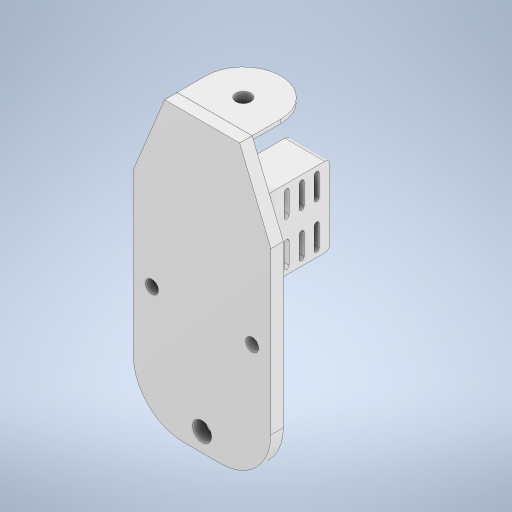
# Autodesk Inventor part: Electromagnet Gantry Plate
Saved by Autodesk Inventor 2023.2 (Build 272271030, 271C)
## iProperties
Created: 2023-04-10
Part Number: Electromagnet Gantry Plate
Material: PC/ABS Plastic
Document SubType Name: Modeling
Designer: ethan
Density: 0.357273 g/cm^3
Appearance: Smooth - White
Author: ethan
Autodesk Inventor part; units mm, degrees
ref_plane "YZ Plane" through (0, 0, 0) normal (1, 0, 0) x (0, 1, 0)
ref_plane "XZ Plane" through (0, 0, 0) normal (0, 1, 0) x (-1, 0, 0)
ref_plane "XY Plane" through (0, 0, 0) normal (0, 0, 1) x (1, 0, 0)
sketch "Sketch1" plane through (0, 0, 0) normal (0, 1, 0) x (-1, 0, 0)
  line L0 (0, 0) -> (55, 0)
  line L1 (55, 0) -> (55, -55)
  line L2 (55, -55) -> (0, -55)
  line L3 (0, -55) -> (0, 0)
  line L4 (47.55, -7.45) -> (7.45, -7.45) construction
  line L5 (7.45, -7.45) -> (7.45, -47.55) construction
  line L6 (7.45, -47.55) -> (47.55, -47.55) construction
  line L7 (47.55, -47.55) -> (47.55, -7.45) construction
  circle A0 centre (47.55, -7.45) radius 2.6
  circle A1 centre (47.55, -47.55) radius 2.6
  circle A2 centre (7.45, -47.55) radius 2.6
  circle A3 centre (7.45, -7.45) radius 2.6
  circle A4 centre (47.55, -7.45) radius 12.5 construction
  circle A5 centre (27.5, -7.45) radius 3.8
  line L8 (55, -55) -> (0, -55)
  line L9 (0, -55) -> (0, -139.9)
  line L10 (0, -139.9) -> (55, -139.9)
  line L11 (55, -139.9) -> (55, -55)
  point P0 (3.72, -55)
  dimension "d0" = 55
  dimension "d1" = 55
  dimension "d2" = 40.1
  dimension "d3" = 40.1
  dimension "d4" = 5.2
  dimension "d5" = 5.2
  dimension "d6" = 5.2
  dimension "d7" = 5.2
  dimension "d8" = 7.45
  dimension "d9" = 7.45
  dimension "d13" = 25
  dimension "d78" = 7.6
  dimension "d160" = 84.9
  constraints: 24 end point, 6 centre point, 6 parallel, 5 coincident, 3 horizontal, 3 perpendicular, 1 midpoint
  measures "d0" distance of L1.end L2.end
  measures "d1" distance of L0.end L1.end
  measures "d2" distance of L6.end L5.end
  measures "d3" distance of L5.end L4.end
  measures "d4" diameter of A0
  measures "d5" diameter of A3
  measures "d6" diameter of A1
  measures "d7" diameter of A2
  measures "d8" distance between parallel lines of L1 L7
  measures "d9" distance from line of L2 L5.end
  measures "d13" diameter of A4
  measures "d78" diameter of A5
  measures "d160" distance of L2.end L9.end
extrude "Extrusion1" add sketch "Sketch1" along normal blind 5 contours L0 L1 L2 L3 | L2 L11 L10 L9 | A0 | A3
fillet "Fillet1" radius 20 2 edges at (-55, 2.5, 0) (0, 2.5, 0)
ref_plane "Work Plane14" through (0, 0, 0) normal (0, 1, 0) x (1, 0, 0)
sketch "Sketch7" plane through (0, 0, 0) normal (0, 1, 0) x (1, 0, 0)
  line L0 (-19.45, 63) -> (-19.45, 55)
  line L1 (-35.55, 19.45) -> (-35.55, 63) projected
  line L2 (-19.45, 55) -> (-35.55, 55)
  line L3 (-35.55, 55) -> (-35.55, 63)
  line L4 (-35.55, 63) -> (-19.45, 63)
  line L5 (-19.45, 63) -> (-19.45, 55)
  circle A0 centre (-47.55, 47.55) radius 2.6 projected
  circle A1 centre (-47.55, 47.55) radius 12
  circle A2 centre (-7.45, 47.55) radius 2.6 projected
  circle A3 centre (-7.45, 47.55) radius 12
  point P0 (0, 0)
  point P1 (-53, 55)
  dimension "d67" = 24
  dimension "d68" = 24
  constraints: 10 end point, 2 centre point, 2 coincident, 2 parallel, 1 horizontal, 1 perpendicular
  measures "d67" diameter of A1
  measures "d68" diameter of A3
extrude "Extrusion9" add sketch "Sketch7" along normal blind 25 contours L0 L2 L1 L4
ref_plane "Work Plane2" through (-19.45, -5, -63) normal (0, 0, -1) x (-1, 0, 0)
sketch "Sketch9" plane through (-19.45, -5, -63) normal (0, 0, -1) x (-1, 0, 0)
  line L0 (0, 0) -> (0, 8) projected
  line L1 (16.1, 8) -> (16.1, 5) projected
  line L2 (0, 8) -> (16.1, 8)
  line L3 (4.55, 8) -> (11.55, 8) projected
  line L4 (8.05, 8) -> (8.05, 21.475)
  circle A0 centre (8.05, 21.475) radius 3
  point P0 (-19.45, 5)
  dimension "d54" = 13.475
  dimension "d55" = 6
  constraints: 4 end point, 1 centre point, 1 coincident, 1 midpoint, 1 perpendicular, 1 vertical
  measures "d54" distance of L4.start L4.end
  measures "d55" diameter of A0
extrude "Extrusion11" cut sketch "Sketch9" against normal through all
ref_plane "Work Plane12" through (-19.45, 0, -63) normal (0, 0, -1) x (-1, 0, 0)
sketch "Sketch10" plane through (-19.45, 0, -63) normal (0, 0, -1) x (-1, 0, 0)
  circle A0 centre (8.05, 16.475) radius 3 projected
  arc A1 (23.05, 16.475) -> (-6.95, 16.475) centre (8.05, 16.475) ccw
  line L0 (-6.95, 16.475) -> (-6.95, 0)
  line L1 (23.05, 16.475) -> (23.05, 0)
  line L2 (-6.95, 0) -> (23.05, 0)
  line L3 (33.55, 0) -> (-17.45, 0) projected
  point P0 (-19.45, 0)
  dimension "d60" = 30
  constraints: 6 end point, 2 point on circle, 2 tangent, 2 vertical, 1 centre point, 1 coincident, 1 collinear
  measures "d60" diameter of A1
extrude "Extrusion12" add sketch "Sketch10" against normal up to surface (8 mm away)
sketch "Sketch18" plane through (0, 5, 0) normal (0, 1, 0) x (1, 0, 0)
  circle A0 centre (-47.55, 47.55) radius 2.6 projected
  circle A1 centre (-47.55, 47.55) radius 12 construction
  line L0 (-47.55, 37.5) -> (0, 37.5)
  line L1 (0, 20) -> (0, 139.9) projected
  line L2 (-47.55, 54.5) -> (0, 54.5)
  line L3 (-47.55, 63) -> (0, 63)
  line L4 (-47.55, 72) -> (0, 72)
  line L5 (-47.55, 80.5) -> (0, 80.5)
  line L6 (-47.55, 139.9) -> (0, 139.9)
  point P0 (0, 0)
  point P1 (0, 63)
  point P2 (0, 83)
  dimension "d106" = 24
  dimension "d107" = 10.05
  dimension "d108" = 17
  dimension "d109" = 8.5
  dimension "d110" = 34.5
  dimension "d111" = 8.5
  dimension "d206" = 102.4
  constraints: 12 end point, 5 parallel, 1 centre point, 1 coincident, 1 horizontal, 1 point on line
  measures "d106" diameter of A1
  measures "d107" distance of A0.centre L0.start
  measures "d108" distance between parallel lines of L0 L2
  measures "d109" distance between parallel lines of L2 L3
  measures "d110" distance between parallel lines of L0 L4
  measures "d111" distance between parallel lines of L4 L5
  measures "d206" distance between parallel lines of L0 L6
ref_plane "Work Plane10" through (-27.5, 0, -20) normal (-1, 0, 0) x (0, 0, 1)
chamfer "Chamfer5" distance 6.5 angle 45 3 edges at (-27.5, 31.475, -55) (-42.5, 10.7375, -55) (-12.5, 10.7375, -55)
chamfer "Chamfer6" distance 6 angle 45 1 edges at (-27.5, 5, -55)
ref_plane "Work Plane16" through (0, 0, -114.9) normal (0, 0, -1) x (-1, 0, 0)
move faces "Move1" translate (0, 0, -51.9) faces at (-27.6205, 7.8323, -63) (-12.6942, 18.8812, -62.5) (-42.5, 8.825, -62.5) (-40.3333, 10.825, -59.3333) (-39.1188, 18.2262, -58.25) (-14.6667, 10.825, -59.3333) (-12.5, 8.825, -62) (-27.6205, 11.8323, -55) (-26.6667, 9, -53) (-30.4903, 16.2336, -57.6667)
sketch "Sketch29" plane through (0, 5, 0) normal (0, 1, 0) x (1, 0, 0)
  line L0 (0, 139.9) -> (-55, 139.9) projected
  line L1 (0, 20) -> (0, 139.9) projected
  line L2 (-55, 139.9) -> (0, 139.9)
  line L3 (0, 139.9) -> (0, 114.877)
  line L4 (0, 114.877) -> (-55, 114.877)
  line L5 (-55, 114.877) -> (-55, 139.9)
  line L6 (-42.5, 114.9) -> (-42.5, 113.4) projected
  line L7 (-50, 84.5) -> (-55, 84.5) projected
  line L8 (-42.5, 114.9) -> (-55, 84.5)
  line L9 (-55, 84.5) -> (-55, 114.877)
  line L10 (-12.5, 114.9) -> (-12.5, 113.4) projected
  line L11 (-12.5, 114.9) -> (0, 84.5)
  line L12 (0, 84.5) -> (0, 114.877)
  line L13 (0, 20) -> (0, 139.9) projected
  point P0 (0, 0)
  point P1 (-42.5, 114.877)
  point P2 (-12.5, 114.877)
  constraints: 16 end point, 2 parallel, 2 perpendicular, 1 collinear, 1 horizontal, 1 point on line
extrude "Extrusion31" cut sketch "Sketch29" against normal through all contours L1 L4 L11 L10 L6 L8 L5 L0 | L1 L11 L4 | L4 L8 L9
sketch "Sketch31" plane through (0, 5, 0) normal (0, 1, 0) x (1, 0, 0)
  circle A0 centre (-47.55, 47.55) radius 2.6 projected
  circle A1 centre (-7.45, 47.55) radius 2.6 projected
  line L0 (-47.55, 47.55) -> (-7.45, 47.55)
  line L1 (-27.5, 47.55) -> (-27.5, 80.5)
  line L2 (-33.5, 47.55) -> (-33.5, 80.5)
  line L3 (-21.5, 47.55) -> (-21.5, 80.5)
  line L4 (-33.5, 80.5) -> (-21.5, 80.5)
  line L5 (-33.5, 47.55) -> (-21.5, 47.55)
  line L6 (-19.5, 84.5) -> (-19.5, 44.7007)
  line L7 (-19.5, 44.7007) -> (-35.5, 44.7007)
  line L8 (-35.5, 44.7007) -> (-35.5, 84.5)
  line L9 (-35.5, 84.5) -> (-19.5, 84.5)
  point P0 (0, 0)
  point P1 (-19.5, 82.5)
  point P2 (-35.5, 81.6507)
  dimension "d216" = 32.95
  dimension "d217" = 6
  dimension "d218" = 6
  dimension "d225" = 2
  dimension "d231" = 4
  constraints: 20 end point, 3 horizontal, 2 parallel, 2 point on line, 1 collinear, 1 midpoint, 1 vertical
  measures "d216" distance of L1.start L1.end
  measures "d217" distance between parallel lines of L1 L2
  measures "d218" distance between parallel lines of L1 L3
  measures "d225" distance between parallel lines of L3 L6
  measures "d231" distance between parallel lines of L4 L9
extrude "Extrusion32" add sketch "Sketch31" along normal blind 38.1 contours L2 L4 L1 L0 | L0 L6 L7 L8 | L0 L8 L9 L6 L3 L4 L2 | L1 L4 L3 L0
sketch "Sketch34" plane through (-35.5, 5, -84.5) normal (-1, 0, 0) x (0, 0, 1)
  line L0 (0, 38.1) -> (39.7993, 38.1) projected
  line L1 (39.7993, 0) -> (39.7993, 38.1) projected
  line L2 (39.7993, 38.1) -> (39.7993, 0)
  line L3 (35.7993, 0) -> (35.7993, 38.1)
  line L4 (28.8493, 0) -> (28.8493, 38.1)
  line L5 (20.3493, 0) -> (20.3493, 38.1)
  line L6 (11.3493, 0) -> (11.3493, 38.1)
  line L7 (2.8493, 0) -> (2.8493, 38.1)
  line L8 (2.8493, 32.8026) -> (11.3493, 32.8026) construction
  line L9 (2.8493, 31.8026) -> (11.3493, 31.8026)
  line L10 (11.3493, 33.8026) -> (2.8493, 33.8026)
  arc A0 (2.8493, 33.8026) -> (2.8493, 31.8026) centre (2.8493, 32.8026) ccw
  arc A1 (11.3493, 31.8026) -> (11.3493, 33.8026) centre (11.3493, 32.8026) ccw
  line L11 (20.3493, 32.8026) -> (28.8493, 32.8026) construction
  line L12 (20.3493, 31.8026) -> (28.8493, 31.8026)
  line L13 (28.8493, 33.8026) -> (20.3493, 33.8026)
  arc A2 (20.3493, 33.8026) -> (20.3493, 31.8026) centre (20.3493, 32.8026) ccw
  arc A3 (28.8493, 31.8026) -> (28.8493, 33.8026) centre (28.8493, 32.8026) ccw
  line L14 (2.8493, 26.8026) -> (28.8493, 26.8026)
  line L15 (2.8493, 20.8026) -> (28.8493, 20.8026)
  line L16 (2.8493, 25.8026) -> (11.3493, 25.8026)
  line L17 (11.3493, 27.8026) -> (2.8493, 27.8026)
  arc A4 (2.8493, 27.8026) -> (2.8493, 25.8026) centre (2.8493, 26.8026) ccw
  arc A5 (11.3493, 25.8026) -> (11.3493, 27.8026) centre (11.3493, 26.8026) ccw
  arc A6 (28.8493, 25.8026) -> (28.8493, 27.8026) centre (28.8493, 26.8026) ccw
  line L18 (20.3493, 25.8026) -> (28.8493, 25.8026)
  line L19 (28.8493, 27.8026) -> (20.3493, 27.8026)
  arc A7 (20.3493, 27.8026) -> (20.3493, 25.8026) centre (20.3493, 26.8026) ccw
  line L20 (2.8493, 19.8026) -> (11.3493, 19.8026)
  line L21 (11.3493, 21.8026) -> (2.8493, 21.8026)
  arc A8 (2.8493, 21.8026) -> (2.8493, 19.8026) centre (2.8493, 20.8026) ccw
  arc A9 (11.3493, 19.8026) -> (11.3493, 21.8026) centre (11.3493, 20.8026) ccw
  arc A10 (28.8493, 19.8026) -> (28.8493, 21.8026) centre (28.8493, 20.8026) ccw
  line L22 (20.3493, 19.8026) -> (28.8493, 19.8026)
  line L23 (28.8493, 21.8026) -> (20.3493, 21.8026)
  arc A11 (20.3493, 21.8026) -> (20.3493, 19.8026) centre (20.3493, 20.8026) ccw
  point P0 (84.5, -5)
  point P1 (7.0993, 32.8026)
  point P2 (24.5993, 32.8026)
  dimension "d232" = 4
  dimension "d233" = 6.95
  dimension "d234" = 8.5
  dimension "d235" = 9
  dimension "d236" = 8.5
  dimension "d237" = 2
  dimension "d238" = 2
  dimension "d239" = 6
  dimension "d240" = 12
  dimension "d241" = 2
  dimension "d242" = 2
  dimension "d243" = 2
  dimension "d244" = 2
  constraints: 48 end point, 24 point on circle, 24 tangent, 12 centre point, 12 equal length, 6 point on line, 3 perpendicular, 2 midpoint
  measures "d232" distance between parallel lines of L1 L3
  measures "d233" distance between parallel lines of L3 L4
  measures "d234" distance between parallel lines of L4 L5
  measures "d235" distance between parallel lines of L5 L6
  measures "d236" distance between parallel lines of L6 L7
  measures "d237" diameter of A1
  measures "d238" diameter of A3
  measures "d239" distance between parallel lines of L8 L14
  measures "d240" distance between parallel lines of L15 L8
  measures "d241" diameter of A5
  measures "d242" diameter of A6
  measures "d243" diameter of A9
  measures "d244" diameter of A10
extrude "Extrusion33" cut sketch "Sketch34" against normal through all contours L10 L6 L9 L7 | L7 A0 | A1 L6 | L13 L4 L12 L5 | L5 A2 | L17 L6 L14 L7 | L7 A4 | A3 L4 | A5 L14 L6 | L14 L6 L16 L7 | L19 L4 L14 L5 | L5 L14 A7 | L14 A5 L6 | L21 L6 L15 L7 | L7 A8 | A6 L4 | L14 L4 L18 L5 | L5 A7 L14 | L15 L6 L20 L7 | A9 L15 L6 | L15 A9 L6 | A10 L4 | L4 L15 L5 L23 | L5 L15 A11 | L15 L5 A11 | L4 L22 L5 L15
sketch "Sketch35" plane through (-35.5, 5, -84.5) normal (-1, 0, 0) x (0, 0, 1)
  line L0 (39.7993, 0) -> (39.7993, 38.1) projected
  line L1 (0, 0) -> (39.7993, 0) projected
  line L2 (39.7993, 38.1) -> (31.6983, 38.1)
  line L3 (31.6983, 38.1) -> (31.6983, 0)
  line L4 (31.6983, 0) -> (39.7993, 0)
  line L5 (39.7993, 0) -> (39.7993, 38.1)
  arc A0 (28.8493, 31.8026) -> (28.8493, 33.8026) centre (28.8493, 32.8026) ccw projected
  point P0 (84.5, -5)
  dimension "d247" = 2.849
  constraints: 8 end point, 2 parallel, 1 horizontal, 1 perpendicular, 1 point on line
  measures "d247" distance from line of A0.centre L3
extrude "Extrusion34" cut sketch "Sketch35" against normal through all
chamfer "Chamfer7" distance 5 angle 45 4 edges at (-35.5, 5, -68.6509) (-27.5, 5, -84.5) (-27.5, 5, -52.8017) (-19.5, 5, -68.6509)
fillet "Fillet16" radius 2 2 edges at (-27.5, 43.1, -52.8017) (-27.5, 43.1, -84.5)
equation "\"d1\" = d0"
equation "\"d3\" = d2"
equation "\"d5\" = d4"
equation "\"d6\" = d4"
equation "\"d7\" = d4"
equation "\"d8\" = -0.5 * d2 + 0.5 * d0"
equation "\"d9\" = -0.5 * d3 + 0.5 * d1"
body "Solid1"
